Autodesk Fusion 360 part; units mm, degrees
(part 5 of 6)
  line L3180 (20.496389, 244.31625) -> (20.214167, 243.716528)
  line L3181 (20.214167, 243.716528) -> (20.0025, 243.116805)
  line L3182 (20.0025, 243.116805) -> (19.861389, 242.446528)
  line L3183 (19.861389, 242.446528) -> (19.790833, 241.811528)
  line L3184 (19.790833, 241.811528) -> (19.755556, 241.14125)
  line L3185 (19.755556, 241.14125) -> (19.790833, 240.50625)
  line L3186 (19.790833, 240.50625) -> (19.861389, 239.835972)
  line L3187 (19.861389, 239.835972) -> (20.0025, 239.200972)
  line L3188 (20.0025, 239.200972) -> (20.214167, 238.60125)
  line L3189 (20.214167, 238.60125) -> (20.496389, 237.96625)
  line L3190 (20.496389, 237.96625) -> (20.813889, 237.401805)
  line L3191 (20.813889, 237.401805) -> (21.166667, 236.872639)
  line L3192 (21.166667, 236.872639) -> (21.59, 236.37875)
  line L3193 (21.59, 236.37875) -> (22.048611, 235.884861)
  line L3194 (22.048611, 235.884861) -> (22.577778, 235.461528)
  line L3195 (22.577778, 235.461528) -> (23.106944, 235.10875)
  line L3196 (23.106944, 235.10875) -> (23.671389, 234.79125)
  line L3197 (23.671389, 234.79125) -> (24.271111, 234.509028)
  line L3198 (24.271111, 234.509028) -> (24.906111, 234.297361)
  line L3199 (24.906111, 234.297361) -> (25.541111, 234.15625)
  line L3200 (25.541111, 234.15625) -> (26.211389, 234.085694)
  line L3201 (26.211389, 234.085694) -> (26.846389, 234.050417)
  line L3202 (26.846389, 234.050417) -> (27.516667, 234.085694)
  line L3203 (27.516667, 234.085694) -> (28.151667, 234.15625)
  line L3204 (28.151667, 234.15625) -> (28.786667, 234.297361)
  line L3205 (28.786667, 234.297361) -> (29.421667, 234.509028)
  line L3206 (29.421667, 234.509028) -> (30.021389, 234.79125)
  line L3207 (30.021389, 234.79125) -> (30.585833, 235.10875)
  line L3208 (30.585833, 235.10875) -> (31.150278, 235.461528)
  line L3209 (31.150278, 235.461528) -> (31.644167, 235.884861)
  line L3210 (31.644167, 235.884861) -> (32.102778, 236.37875)
  line L3211 (32.102778, 236.37875) -> (32.526111, 236.872639)
  line L3212 (32.526111, 236.872639) -> (32.914167, 237.401805)
  line L3213 (32.914167, 237.401805) -> (33.231667, 237.96625)
  line L3214 (33.231667, 237.96625) -> (33.478611, 238.60125)
  line L3215 (33.478611, 238.60125) -> (33.690278, 239.200972)
  line L3216 (33.690278, 239.200972) -> (33.831389, 239.835972)
  line L3217 (33.831389, 239.835972) -> (33.937222, 240.50625)
  line L3218 (33.937222, 240.50625) -> (33.9725, 241.14125)
  line L3219 (28.116389, 289.577639) -> (28.116389, 289.471805)
  line L3220 (7.3025, 233.52125) -> (7.337778, 233.909305)
  line L3221 (31.326667, 225.760139) -> (29.845, 225.760139)
  line L3222 (9.419167, 223.467083) -> (9.454444, 223.220139)
  line L3223 (24.518056, 229.07625) -> (24.518056, 228.970417)
  line L3224 (24.518056, 228.970417) -> (24.482778, 228.899861)
  line L3225 (22.5425, 223.290694) -> (22.789444, 223.467083)
  line L3226 (39.722778, 242.72875) -> (39.863889, 242.446528)
  line L3227 (39.863889, 242.446528) -> (39.899167, 242.234861)
  line L3228 (39.511111, 242.834583) -> (39.616944, 242.799305)
  line L3229 (39.616944, 242.799305) -> (39.722778, 242.72875)
  line L3230 (24.765, 228.723472) -> (24.835556, 228.75875)
  line L3231 (24.835556, 228.75875) -> (24.870833, 228.794028)
  line L3232 (25.964444, 287.390417) -> (26.916944, 285.767639)
  line L3233 (22.789444, 223.467083) -> (22.965833, 223.643472)
  line L3234 (20.743333, 223.749305) -> (20.990278, 223.467083)
  line L3235 (23.318611, 230.593194) -> (23.565556, 230.487361)
  line L3236 (23.565556, 230.487361) -> (23.777222, 230.310972)
  line L3237 (23.777222, 230.310972) -> (23.918333, 229.993472)
  line L3238 (23.389167, 231.475139) -> (23.283333, 231.580972)
  line L3239 (23.283333, 231.580972) -> (23.106944, 231.61625)
  line L3240 (23.106944, 231.61625) -> (22.895278, 231.61625)
  line L3241 (40.005, 232.25125) -> (39.6875, 232.427639)
  line L3242 (16.721667, 291.024028) -> (16.474722, 291.094583)
  line L3243 (16.474722, 291.094583) -> (16.227778, 291.129861)
  line L3244 (38.205833, 233.168472) -> (38.205833, 236.343472)
  line L3245 (5.856111, 223.467083) -> (5.856111, 227.030139)
  line L3246 (5.856111, 227.030139) -> (5.856111, 227.17125)
  line L3247 (39.0525, 250.877917) -> (39.123056, 250.807361)
  line L3248 (39.123056, 250.807361) -> (39.158333, 250.772083)
  line L3249 (39.158333, 250.772083) -> (39.228889, 250.736805)
  line L3250 (39.228889, 250.736805) -> (39.299444, 250.736805)
  line L3251 (38.558611, 251.93625) -> (39.0525, 250.877917)
  line L3252 (39.440556, 265.306528) -> (39.37, 265.165417)
  line L3253 (38.205833, 236.343472) -> (38.205833, 236.449305)
  line L3254 (38.276389, 291.129861) -> (38.241111, 291.094583)
  line L3255 (40.005, 249.71375) -> (40.005, 251.93625)
  line L3256 (40.463611, 252.959305) -> (40.463611, 249.71375)
  line L3257 (30.938611, 291.059305) -> (30.903333, 291.129861)
  line L3258 (40.040278, 243.787083) -> (39.934444, 243.822361)
  line L3259 (39.828611, 241.917361) -> (39.899167, 242.234861)
  line L3260 (41.627778, 263.013472) -> (41.733611, 263.013472)
  line L3261 (41.380833, 263.295694) -> (41.416111, 263.119305)
  line L3262 (38.840833, 243.575417) -> (38.946667, 243.469583)
  line L3263 (27.340278, 291.129861) -> (27.305, 291.200417)
  line L3264 (17.250833, 222.549861) -> (22.154444, 222.549861)
  line L3265 (15.804444, 222.549861) -> (11.324167, 218.034306)
  line L3266 (40.287222, 262.378472) -> (40.181389, 262.801805)
  line L3267 (42.298056, 264.248194) -> (42.2275, 264.248194)
  line L3268 (37.994167, 291.588472) -> (38.064722, 291.553194)
  line L3269 (40.357778, 242.234861) -> (40.3225, 241.882083)
  line L3270 (20.778611, 225.548472) -> (20.743333, 225.26625)
  line L3271 (22.013333, 225.548472) -> (21.942778, 225.513194)
  line L3272 (22.754167, 225.548472) -> (22.154444, 225.548472)
  line L3273 (37.394444, 293.175972) -> (35.983333, 293.175972)
  line L3274 (24.835556, 285.59125) -> (24.906111, 285.626528)
  line L3275 (24.482778, 285.802917) -> (24.482778, 285.697083)
  line L3276 (35.983333, 293.175972) -> (35.983333, 291.588472)
  line L3277 (22.119167, 225.019305) -> (22.013333, 225.019305)
  line L3278 (39.193611, 276.736528) -> (39.264167, 276.665972)
  line L3279 (35.736389, 226.924305) -> (35.665833, 226.889028)
  line L3280 (39.698083, 284.522333) -> (36.935833, 281.745972)
  line L3281 (30.1625, 295.045694) -> (30.1625, 294.939861)
  line L3282 (38.205833, 242.164305) -> (38.241111, 242.340694)
  line L3283 (38.311667, 294.904583) -> (38.276389, 294.869305)
  line L3284 (37.711944, 223.220139) -> (37.676667, 223.290694)
  line L3285 (39.334722, 295.43375) -> (39.722778, 295.821805)
  line L3286 (26.881667, 252.077361) -> (26.387778, 252.077361)
  line L3287 (35.454167, 262.378472) -> (34.925, 264.212917)
  line L3288 (34.925, 264.212917) -> (34.360556, 262.378472)
  line L3289 (34.360556, 262.378472) -> (35.454167, 262.378472)
  line L3290 (32.102778, 227.347639) -> (32.138056, 227.277083)
  line L3291 (35.348333, 285.873472) -> (35.348333, 289.507083)
  line L3292 (15.663333, 286.86125) -> (16.051389, 286.825972)
  line L3293 (17.78, 290.283194) -> (17.603611, 290.459583)
  line L3294 (38.170556, 289.789305) -> (38.205833, 289.754028)
  line L3295 (21.096111, 289.789305) -> (20.955, 289.71875)
  line L3296 (20.955, 289.71875) -> (20.919722, 289.612917)
  line L3297 (20.073056, 290.283194) -> (25.611667, 295.821805)
  line L3298 (15.980833, 291.129861) -> (15.5575, 291.059305)
  line L3299 (16.227778, 291.129861) -> (15.980833, 291.129861)
  line L3300 (25.611667, 295.821805) -> (20.672778, 295.821805)
  line L3301 (17.603611, 290.459583) -> (17.391944, 290.635972)
  line L3302 (17.391944, 290.635972) -> (17.215556, 290.812361)
  line L3303 (29.068889, 231.722083) -> (28.998333, 231.651528)
  line L3304 (32.208611, 223.255417) -> (32.173333, 223.220139)
  line L3305 (37.641389, 293.669861) -> (37.711944, 293.599305)
  line L3306 (38.1, 252.924028) -> (38.135278, 253.100417)
  line L3307 (32.914167, 237.401805) -> (33.231667, 237.96625)
  line L3308 (33.231667, 237.96625) -> (33.478611, 238.60125)
  line L3309 (38.346944, 291.376805) -> (38.346944, 291.30625)
  line L3310 (31.891111, 227.382917) -> (32.102778, 227.347639)
  line L3311 (29.668611, 227.382917) -> (31.891111, 227.382917)
  line L3312 (32.208611, 227.100694) -> (32.173333, 226.994861)
  line L3313 (13.899444, 280.440694) -> (14.181667, 280.581805)
  line L3314 (31.538333, 280.440694) -> (31.785278, 280.264305)
  line L3315 (38.170556, 226.85375) -> (38.170556, 223.431805)
  line L3316 (38.205833, 233.027361) -> (38.205833, 233.168472)
  line L3317 (42.368611, 263.542639) -> (42.474444, 263.507361)
  line L3318 (19.861389, 239.835972) -> (20.0025, 239.200972)
  line L3319 (20.0025, 239.200972) -> (20.214167, 238.60125)
  line L3320 (32.208611, 223.467083) -> (32.243889, 223.396528)
  line L3321 (39.299444, 250.736805) -> (39.228889, 250.736805)
  line L3322 (20.955, 289.71875) -> (21.096111, 289.789305)
  line L3323 (21.096111, 289.789305) -> (21.2725, 289.824583)
  line L3324 (21.2725, 289.824583) -> (23.459722, 289.824583)
  line L3325 (22.471944, 229.71125) -> (22.436667, 229.817083)
  line L3326 (22.436667, 229.817083) -> (22.366111, 229.852361)
  line L3327 (38.629167, 243.116805) -> (38.488056, 243.257917)
  line L3328 (34.748611, 294.445972) -> (34.572222, 294.763472)
  line L3329 (19.05, 226.148194) -> (19.014722, 225.936528)
  line L3330 (22.013333, 225.548472) -> (22.154444, 225.548472)
  line L3331 (39.758056, 246.397639) -> (39.264167, 248.020417)
  line L3332 (39.264167, 248.020417) -> (38.770278, 246.397639)
  line L3333 (38.770278, 246.397639) -> (39.758056, 246.397639)
  line L3334 (23.847778, 246.750417) -> (24.412222, 247.032639)
  line L3335 (40.357778, 233.097917) -> (40.357778, 232.992083)
  line L3336 (27.410833, 291.094583) -> (27.340278, 291.129861)
  line L3337 (32.138056, 227.277083) -> (32.208611, 227.206528)
  line L3338 (40.463611, 253.100417) -> (40.463611, 252.959305)
  line L3339 (32.914167, 244.880694) -> (32.526111, 245.445139)
  line L3340 (32.526111, 245.445139) -> (32.102778, 245.939028)
  line L3341 (30.973889, 280.687639) -> (31.291389, 280.581805)
  line L3342 (39.123056, 265.694583) -> (39.228889, 265.694583)
  line L3343 (31.538333, 257.157361) -> (31.291389, 257.01625)
  line L3344 (32.138056, 226.924305) -> (32.102778, 226.889028)
  line L3345 (32.208611, 258.180417) -> (32.138056, 257.898194)
  line L3346 (14.181667, 257.01625) -> (13.899444, 257.157361)
  line L3347 (29.315833, 227.17125) -> (29.386389, 227.277083)
  line L3348 (31.291389, 225.26625) -> (29.845, 225.26625)
  line L3349 (39.017222, 237.33125) -> (39.017222, 237.190139)
  line L3350 (39.017222, 237.190139) -> (39.0525, 237.154861)
  line L3351 (33.901944, 286.261528) -> (34.043056, 286.402639)
  line L3352 (34.043056, 286.402639) -> (34.078333, 286.579028)
  line L3353 (20.990278, 238.707083) -> (21.2725, 238.177917)
  line L3354 (21.2725, 238.177917) -> (21.59, 237.613472)
  line L3355 (39.37, 244.457361) -> (39.123056, 244.457361)
  line L3356 (39.722778, 295.821805) -> (43.991389, 295.821805)
  line L3357 (29.950833, 253.488472) -> (29.280556, 252.112639)
  line L3358 (30.127222, 253.594305) -> (30.056667, 253.594305)
  line L3359 (28.398611, 233.450694) -> (29.104167, 233.591805)
  line L3360 (36.794722, 272.503194) -> (36.83, 272.57375)
  line L3361 (28.186944, 289.71875) -> (28.222222, 289.754028)
  line L3362 (35.806944, 289.507083) -> (35.806944, 288.166528)
  line L3363 (40.357778, 236.414028) -> (40.3225, 236.308194)
  line L3364 (36.83, 272.397361) -> (36.794722, 272.503194)
  line L3365 (13.6525, 257.369028) -> (13.476111, 257.615972)
  line L3366 (38.770278, 241.77625) -> (38.911389, 241.635139)
  line L3367 (35.736389, 289.754028) -> (35.806944, 289.648194)
  line L3368 (40.393056, 253.170972) -> (40.463611, 253.100417)
  line L3369 (29.280556, 252.112639) -> (29.950833, 253.488472)
  line L3370 (38.276389, 232.921528) -> (38.382222, 232.88625)
  line L3371 (38.382222, 232.88625) -> (38.488056, 232.88625)
  line L3372 (38.205833, 236.343472) -> (38.205833, 233.168472)
  line L3373 (38.523333, 236.660972) -> (38.382222, 236.625694)
  line L3374 (38.382222, 236.625694) -> (38.241111, 236.555139)
  line L3375 (29.986111, 230.381528) -> (29.986111, 229.111528)
  line L3376 (20.496389, 241.14125) -> (20.531667, 240.541528)
  line L3377 (20.531667, 240.541528) -> (20.6375, 239.906528)
  line L3378 (37.958889, 289.789305) -> (38.064722, 289.824583)
  line L3379 (30.832778, 294.975139) -> (30.832778, 291.341528)
  line L3380 (31.538333, 225.724861) -> (31.608889, 225.689583)
  line L3381 (14.499167, 280.687639) -> (14.781389, 280.722917)
  line L3382 (1.446389, 284.709305) -> (1.446389, 284.391805)
  line L3383 (5.150556, 292.999583) -> (1.446389, 284.709305)
  line L3384 (21.942778, 245.198194) -> (22.366111, 245.656805)
  line L3385 (40.3225, 228.970417) -> (40.3225, 228.899861)
  line L3386 (40.3225, 228.899861) -> (40.251944, 228.829305)
  line L3387 (40.251944, 228.829305) -> (40.181389, 228.75875)
  line L3388 (40.181389, 228.75875) -> (40.075556, 228.75875)
  line L3389 (40.075556, 228.75875) -> (39.969722, 228.75875)
  line L3390 (39.969722, 228.75875) -> (39.934444, 228.794028)
  line L3391 (39.934444, 228.794028) -> (39.899167, 228.864583)
  line L3392 (39.899167, 228.864583) -> (39.0525, 230.310972)
  line L3393 (39.0525, 230.310972) -> (38.735, 230.310972)
  line L3394 (38.735, 230.310972) -> (38.735, 229.040972)
  line L3395 (38.735, 229.040972) -> (38.735, 228.935139)
  line L3396 (38.735, 228.935139) -> (38.699722, 228.829305)
  line L3397 (38.699722, 228.829305) -> (38.664444, 228.75875)
  line L3398 (38.664444, 228.75875) -> (38.593889, 228.75875)
  line L3399 (38.593889, 228.75875) -> (38.488056, 228.723472)
  line L3400 (38.488056, 228.723472) -> (38.4175, 228.75875)
  line L3401 (38.4175, 228.75875) -> (38.311667, 228.794028)
  line L3402 (38.311667, 228.794028) -> (38.276389, 228.864583)
  line L3403 (38.276389, 228.864583) -> (38.276389, 228.899861)
  line L3404 (38.276389, 228.899861) -> (38.276389, 229.040972)
  line L3405 (38.276389, 229.040972) -> (38.276389, 232.180694)
  line L3406 (38.276389, 232.180694) -> (38.276389, 232.286528)
  line L3407 (38.276389, 232.286528) -> (38.311667, 232.392361)
  line L3408 (38.311667, 232.392361) -> (38.452778, 232.498194)
  line L3409 (38.452778, 232.498194) -> (38.593889, 232.498194)
  line L3410 (38.593889, 232.498194) -> (39.334722, 232.498194)
  line L3411 (39.334722, 232.498194) -> (39.6875, 232.427639)
  line L3412 (39.6875, 232.427639) -> (40.005, 232.25125)
  line L3413 (40.005, 232.25125) -> (40.216667, 231.863194)
  line L3414 (40.216667, 231.863194) -> (40.3225, 231.404583)
  line L3415 (40.3225, 231.404583) -> (40.287222, 231.122361)
  line L3416 (40.287222, 231.122361) -> (40.181389, 230.840139)
  line L3417 (40.181389, 230.840139) -> (39.934444, 230.522639)
  line L3418 (39.934444, 230.522639) -> (39.616944, 230.34625)
  line L3419 (39.616944, 230.34625) -> (39.581667, 230.310972)
  line L3420 (39.581667, 230.310972) -> (40.216667, 229.182083)
  line L3421 (40.216667, 229.182083) -> (40.251944, 229.146805)
  line L3422 (40.251944, 229.146805) -> (40.287222, 229.07625)
  line L3423 (40.287222, 229.07625) -> (40.3225, 229.040972)
  line L3424 (40.3225, 229.040972) -> (40.3225, 228.970417)
  line L3425 (38.488056, 232.88625) -> (38.382222, 232.88625)
  line L3426 (38.382222, 232.88625) -> (38.276389, 232.921528)
  line L3427 (13.229167, 279.452917) -> (13.335, 279.735139)
  line L3428 (15.24, 225.760139) -> (15.451667, 225.724861)
  line L3429 (40.040278, 232.88625) -> (38.488056, 232.88625)
  line L3430 (42.403889, 264.283472) -> (42.298056, 264.248194)
  line L3431 (14.181667, 280.581805) -> (14.499167, 280.687639)
  line L3432 (15.522222, 225.689583) -> (15.5575, 225.58375)
  line L3433 (31.150278, 235.461528) -> (31.644167, 235.884861)
  line L3434 (31.644167, 235.884861) -> (32.102778, 236.37875)
  line L3435 (27.410833, 285.661805) -> (27.305, 285.59125)
  line L3436 (21.872222, 225.054583) -> (21.801667, 225.125139)
  line L3437 (32.949444, 243.010972) -> (33.090556, 242.375972)
  line L3438 (13.6525, 280.264305) -> (13.899444, 280.440694)
  line L3439 (32.0675, 223.643472) -> (32.173333, 223.537639)
  line L3440 (35.418889, 285.626528) -> (35.348333, 285.732361)
  line L3441 (35.806944, 287.707917) -> (35.806944, 285.873472)
  line L3442 (41.169167, 261.814028) -> (41.310278, 261.708194)
  line L3443 (39.264167, 248.020417) -> (39.758056, 246.397639)
  line L3444 (39.405278, 244.95125) -> (39.440556, 244.95125)
  line L3445 (22.789444, 226.254028) -> (22.718889, 226.289305)
  line L3446 (20.849167, 225.830694) -> (21.060833, 226.254028)
  line L3447 (21.201944, 223.99625) -> (20.990278, 224.31375)
  line L3448 (20.990278, 224.31375) -> (20.849167, 224.666528)
  line L3449 (28.786667, 247.985139) -> (28.151667, 248.161528)
  line L3450 (28.151667, 248.161528) -> (27.516667, 248.232083)
  line L3451 (39.264167, 276.524861) -> (39.228889, 276.419028)
  line L3452 (39.228889, 250.736805) -> (39.158333, 250.772083)
  line L3453 (33.725556, 284.885694) -> (30.585833, 281.745972)
  line L3454 (38.311667, 232.392361) -> (38.276389, 232.286528)
  line L3455 (37.641389, 293.669861) -> (37.429722, 293.705139)
  line L3456 (37.394444, 293.175972) -> (37.641389, 293.21125)
  line L3457 (37.641389, 293.21125) -> (37.711944, 293.246528)
  line L3458 (31.467778, 228.829305) -> (31.4325, 228.75875)
  line L3459 (13.899444, 289.048472) -> (13.934722, 288.695694)
  line L3460 (13.934722, 288.695694) -> (14.005278, 288.307639)
  line L3461 (30.021389, 247.526528) -> (29.421667, 247.773472)
  line L3462 (29.421667, 247.773472) -> (28.786667, 247.985139)
  line L3463 (19.332222, 226.85375) -> (19.085278, 227.135972)
  line L3464 (19.085278, 227.135972) -> (18.697222, 227.312361)
  line L3465 (39.6875, 241.211805) -> (39.969722, 241.352917)
  line L3466 (39.969722, 241.352917) -> (40.181389, 241.564583)
  line L3467 (40.181389, 241.564583) -> (40.3225, 241.882083)
  line L3468 (40.3225, 241.882083) -> (40.357778, 242.234861)
  line L3469 (8.713611, 223.220139) -> (8.748889, 223.255417)
  line L3470 (8.748889, 223.255417) -> (8.748889, 223.396528)
  line L3471 (17.250833, 222.549861) -> (22.154444, 222.549861)
  line L3472 (23.600833, 222.549861) -> (28.504444, 222.549861)
  line L3473 (29.950833, 222.549861) -> (31.855833, 222.549861)
  line L3474 (38.135278, 249.537361) -> (38.1, 249.749028)
  line L3475 (8.396111, 223.114305) -> (8.643056, 223.149583)
  line L3476 (8.643056, 223.149583) -> (8.713611, 223.220139)
  line L3477 (30.903333, 291.129861) -> (30.832778, 291.165139)
  line L3478 (24.906111, 247.985139) -> (24.271111, 247.773472)
  line L3479 (24.271111, 247.773472) -> (23.671389, 247.526528)
  line L3480 (40.3225, 241.882083) -> (40.181389, 241.564583)
  line L3481 (29.315833, 223.467083) -> (29.315833, 227.030139)
  line L3482 (40.357778, 233.168472) -> (40.357778, 233.097917)
  line L3483 (17.321389, 226.85375) -> (18.273889, 226.85375)
  line L3484 (17.321389, 225.407361) -> (17.321389, 226.85375)
  line L3485 (11.43, 232.639305) -> (11.535833, 232.992083)
  line L3486 (11.535833, 232.992083) -> (11.606389, 233.344861)
  line L3487 (23.988889, 229.640694) -> (23.918333, 229.993472)
  line L3488 (28.716111, 230.628472) -> (28.680833, 230.699028)
  line L3489 (28.680833, 230.699028) -> (28.645556, 230.734305)
  line L3490 (28.645556, 230.734305) -> (28.469167, 230.769583)
  line L3491 (27.093333, 251.689305) -> (27.128611, 251.724583)
  line L3492 (27.693056, 250.701528) -> (27.093333, 251.689305)
  line L3493 (27.375556, 284.885694) -> (27.199167, 284.885694)
  line L3494 (38.170556, 289.789305) -> (38.064722, 289.824583)
  line L3495 (38.276389, 285.873472) -> (38.276389, 289.507083)
  line L3496 (38.064722, 285.555972) -> (38.170556, 285.59125)
  line L3497 (31.573611, 247.455972) -> (31.009167, 247.844028)
  line L3498 (31.009167, 247.844028) -> (30.374167, 248.196805)
  line L3499 (8.713611, 223.537639) -> (8.5725, 223.643472)
  line L3500 (33.090556, 242.375972) -> (33.161111, 241.77625)
  line L3501 (32.173333, 226.994861) -> (32.138056, 226.924305)
  line L3502 (25.611667, 247.385417) -> (26.246667, 247.455972)
  line L3503 (19.508611, 225.760139) -> (19.579167, 226.148194)
  line L3504 (19.473333, 223.608194) -> (18.520833, 224.913472)
  line L3505 (11.606389, 233.344861) -> (11.535833, 232.992083)
  line L3506 (32.243889, 223.396528) -> (32.208611, 223.255417)
  line L3507 (38.064722, 223.149583) -> (37.923611, 223.114305)
  line L3508 (26.281944, 287.884305) -> (27.093333, 289.365972)
  line L3509 (29.5275, 227.347639) -> (29.668611, 227.382917)
  line L3510 (28.645556, 230.381528) -> (28.433889, 230.381528)
  line L3511 (34.219444, 288.730972) -> (34.29, 288.695694)
  line L3512 (34.29, 288.695694) -> (34.360556, 288.695694)
  line L3513 (27.340278, 228.723472) -> (27.410833, 228.723472)
  line L3514 (29.068889, 231.792639) -> (29.033611, 231.898472)
  line L3515 (29.033611, 231.898472) -> (28.963056, 231.969028)
  line L3516 (28.963056, 231.969028) -> (28.821944, 232.004305)
  line L3517 (28.292778, 253.488472) -> (28.328056, 253.559028)
  line L3518 (22.401389, 223.819861) -> (22.507222, 223.960972)
  line L3519 (31.361944, 236.660972) -> (30.868056, 236.237639)
  line L3520 (27.234444, 231.93375) -> (27.199167, 231.827917)
  line L3521 (27.199167, 231.827917) -> (27.199167, 231.722083)
  line L3522 (28.821944, 232.004305) -> (27.481389, 232.004305)
  line L3523 (13.193889, 279.135417) -> (13.229167, 279.452917)
  line L3524 (18.803056, 226.677361) -> (18.944167, 226.500972)
  line L3525 (18.944167, 226.500972) -> (19.014722, 226.324583)
  line L3526 (32.737778, 243.575417) -> (32.455556, 244.139861)
  line L3527 (32.455556, 244.139861) -> (32.138056, 244.669028)
  line L3528 (13.476111, 280.017361) -> (13.6525, 280.264305)
  line L3529 (32.984722, 227.312361) -> (33.231667, 227.382917)
  line L3530 (35.771667, 227.100694) -> (35.771667, 227.030139)
  line L3531 (39.37, 265.165417) -> (37.500278, 261.284861)
  line L3532 (29.598056, 228.970417) -> (29.598056, 231.757361)
  line L3533 (28.222222, 227.312361) -> (28.292778, 227.347639)
  line L3534 (16.051389, 226.924305) -> (16.016111, 226.889028)
  line L3535 (32.138056, 279.735139) -> (32.208611, 279.452917)
  line L3536 (8.607778, 227.347639) -> (8.396111, 227.382917)
  line L3537 (23.777222, 285.626528) -> (23.8125, 285.697083)
  line L3538 (21.237222, 285.555972) -> (23.459722, 285.555972)
  line L3539 (29.386389, 227.277083) -> (29.5275, 227.347639)
  line L3540 (38.770278, 244.210417) -> (38.911389, 244.386805)
  line L3541 (30.973889, 256.945694) -> (30.656389, 256.910417)
  line L3542 (41.768889, 261.708194) -> (41.557222, 261.672917)
  line L3543 (28.081111, 234.932361) -> (28.716111, 235.073472)
  line L3544 (28.716111, 235.073472) -> (29.280556, 235.285139)
  line L3545 (38.593889, 242.41125) -> (38.664444, 242.305417)
  line L3546 (25.294167, 289.612917) -> (25.964444, 288.44875)
  line L3547 (32.208611, 279.452917) -> (32.243889, 279.135417)
  line L3548 (31.538333, 225.301528) -> (31.291389, 225.26625)
  line L3549 (27.798889, 294.763472) -> (27.798889, 293.705139)
  line L3550 (37.676667, 226.85375) -> (36.794722, 226.85375)
  line L3551 (40.3225, 232.956805) -> (40.287222, 232.921528)
  line L3552 (32.102778, 223.149583) -> (31.855833, 223.114305)
  line L3553 (39.793333, 244.845417) -> (39.616944, 244.915972)
  line L3554 (28.680833, 227.135972) -> (28.680833, 227.030139)
  line L3555 (1.446389, 284.391805) -> (1.446389, 284.709305)
  line L3556 (21.2725, 238.177917) -> (20.990278, 238.707083)
  line L3557 (42.545, 263.189861) -> (42.545, 262.202083)
  line L3558 (21.942778, 237.119583) -> (21.59, 237.613472)
  line L3559 (32.455556, 244.139861) -> (32.737778, 243.575417)
  line L3560 (36.794722, 226.85375) -> (36.583056, 226.889028)
  line L3561 (13.758333, 226.85375) -> (13.758333, 225.760139)
  line L3562 (28.010556, 224.137361) -> (28.116389, 224.419583)
  line L3563 (36.300833, 222.549861) -> (37.923611, 222.549861)
  line L3564 (37.923611, 222.549861) -> (41.204444, 222.549861)
  line L3565 (27.6225, 230.381528) -> (27.6225, 228.970417)
  line L3566 (28.610278, 227.312361) -> (28.645556, 227.206528)
  line L3567 (22.577778, 225.019305) -> (22.119167, 225.019305)
  line L3568 (13.758333, 225.760139) -> (15.24, 225.760139)
  line L3569 (38.382222, 243.434305) -> (38.488056, 243.257917)
  line L3570 (39.405278, 241.14125) -> (39.123056, 241.14125)
  line L3571 (34.466389, 289.330694) -> (34.219444, 289.542361)
  line L3572 (34.219444, 289.542361) -> (33.901944, 289.71875)
  line L3573 (22.824722, 246.080139) -> (23.318611, 246.432917)
  line L3574 (28.292778, 250.384028) -> (28.2575, 250.560417)
  line L3575 (22.154444, 231.157639) -> (22.189722, 230.910694)
  line L3576 (22.189722, 230.910694) -> (22.260278, 230.699028)
  line L3577 (32.208611, 289.119028) -> (32.596667, 289.542361)
  line L3578 (32.596667, 289.542361) -> (32.949444, 289.71875)
  line L3579 (32.737778, 243.575417) -> (32.949444, 243.010972)
  line L3580 (29.5275, 223.114305) -> (29.421667, 223.184861)
  line L3581 (20.6375, 239.906528) -> (20.531667, 240.541528)
  line L3582 (31.996944, 280.017361) -> (32.138056, 279.735139)
  line L3583 (31.785278, 280.264305) -> (31.996944, 280.017361)
  line L3584 (29.315833, 227.030139) -> (29.315833, 227.17125)
  line L3585 (13.476111, 280.017361) -> (13.335, 279.735139)
  line L3586 (13.335, 279.735139) -> (13.229167, 279.452917)
  line L3587 (13.229167, 279.452917) -> (13.193889, 279.135417)
  line L3588 (30.656389, 280.722917) -> (14.781389, 280.722917)
  line L3589 (39.722778, 242.72875) -> (39.616944, 242.799305)
  line L3590 (35.806944, 288.166528) -> (37.817778, 288.166528)
  line L3591 (16.086667, 227.277083) -> (16.121944, 227.206528)
  line L3592 (32.173333, 223.220139) -> (32.102778, 223.149583)
  line L3593 (29.668611, 223.114305) -> (29.5275, 223.114305)
  line L3594 (32.208611, 227.135972) -> (32.208611, 227.100694)
  line L3595 (31.855833, 223.114305) -> (29.668611, 223.114305)
  line L3596 (41.521944, 263.507361) -> (41.627778, 263.542639)
  line L3597 (41.416111, 263.119305) -> (41.380833, 263.295694)
  line L3598 (39.37, 226.994861) -> (39.334722, 226.924305)
  line L3599 (35.489444, 289.789305) -> (35.56, 289.824583)
  line L3600 (29.245278, 293.705139) -> (29.386389, 293.705139)
  line L3601 (31.785278, 287.249305) -> (31.75, 287.672639)
  line L3602 (31.75, 287.672639) -> (31.785278, 288.13125)
  line L3603 (35.665833, 285.555972) -> (35.595278, 285.555972)
  line L3604 (38.170556, 223.255417) -> (38.064722, 223.149583)
  line L3605 (29.492222, 293.634583) -> (29.5275, 293.599305)
  line L3606 (40.287222, 240.400417) -> (40.181389, 240.329861)
  line L3607 (26.140833, 224.878194) -> (26.176111, 224.772361)
  line L3608 (27.551944, 228.75875) -> (27.516667, 228.723472)
  line L3609 (29.739167, 232.004305) -> (29.845, 232.004305)
  line L3610 (6.0325, 227.347639) -> (6.208889, 227.382917)
  line L3611 (6.208889, 227.382917) -> (8.396111, 227.382917)
  line L3612 (40.3225, 232.956805) -> (40.357778, 232.992083)
  line L3613 (40.357778, 232.992083) -> (40.357778, 233.097917)
  line L3614 (38.488056, 232.88625) -> (40.040278, 232.88625)
  line L3615 (24.553333, 285.626528) -> (24.482778, 285.697083)
  line L3616 (29.068889, 231.792639) -> (29.068889, 231.722083)
  line L3617 (34.748611, 291.482639) -> (34.713333, 291.517917)
  line L3618 (34.819167, 291.30625) -> (34.783889, 291.412083)
  line L3619 (34.783889, 291.412083) -> (34.748611, 291.482639)
  line L3620 (38.735, 230.310972) -> (39.0525, 230.310972)
  line L3621 (38.735, 229.040972) -> (38.735, 230.310972)
  line L3622 (39.158333, 237.01375) -> (39.087778, 237.084305)
  line L3623 (38.770278, 241.211805) -> (38.488056, 241.388194)
  line L3624 (15.204722, 225.26625) -> (13.758333, 225.26625)
  line L3625 (25.999722, 229.675972) -> (25.576389, 231.087083)
  line L3626 (25.576389, 231.087083) -> (25.153056, 229.675972)
  line L3627 (25.153056, 229.675972) -> (25.999722, 229.675972)
  line L3628 (14.640278, 287.355139) -> (14.957778, 287.108194)
  line L3629 (32.385, 291.059305) -> (32.455556, 291.094583)
  line L3630 (32.455556, 291.094583) -> (32.490833, 291.165139)
  line L3631 (21.343056, 246.785694) -> (20.884444, 246.291805)
  line L3632 (20.884444, 246.291805) -> (20.461111, 245.727361)
  line L3633 (20.461111, 245.727361) -> (20.073056, 245.127639)
  line L3634 (35.806944, 288.166528) -> (35.806944, 289.507083)
  line L3635 (37.817778, 288.166528) -> (35.806944, 288.166528)
  line L3636 (25.505833, 232.004305) -> (25.435278, 231.969028)
  line L3637 (25.435278, 231.969028) -> (25.4, 231.93375)
  line L3638 (28.927778, 231.61625) -> (28.821944, 231.61625)
  line L3639 (34.536944, 287.919583) -> (34.6075, 287.778472)
  line L3640 (39.334722, 289.08375) -> (39.334722, 284.885694)
  line L3641 (27.093333, 289.365972) -> (26.281944, 287.884305)
  line L3642 (27.693056, 253.029861) -> (27.481389, 253.382639)
  line L3643 (27.481389, 253.382639) -> (27.199167, 253.559028)
  line L3644 (40.216667, 243.892917) -> (40.251944, 243.963472)
  line L3645 (40.251944, 243.963472) -> (40.287222, 244.034028)
  line L3646 (39.828611, 243.892917) -> (39.899167, 243.857639)
  line L3647 (39.899167, 243.857639) -> (39.934444, 243.822361)
  line L3648 (33.655, 287.460972) -> (34.113611, 287.460972)
  line L3649 (33.408056, 287.49625) -> (33.478611, 287.460972)
  line L3650 (31.926389, 288.589861) -> (31.785278, 288.13125)
  line L3651 (31.785278, 288.13125) -> (31.75, 287.672639)
  line L3652 (41.733611, 263.013472) -> (41.627778, 263.013472)
  line L3653 (15.663333, 286.86125) -> (16.051389, 286.825972)
  line L3654 (26.035, 224.984028) -> (26.105556, 224.94875)
  line L3655 (13.758333, 226.85375) -> (15.769167, 226.85375)
  line L3656 (13.758333, 225.760139) -> (13.758333, 226.85375)
  line L3657 (15.24, 225.760139) -> (13.758333, 225.760139)
  line L3658 (13.193889, 279.135417) -> (13.193889, 258.497917)
  line L3659 (17.674167, 218.034306) -> (12.735278, 218.034306)
  line L3660 (12.735278, 218.034306) -> (17.250833, 222.549861)
  line L3661 (21.448889, 286.085139) -> (21.448889, 287.707917)
  line L3662 (27.551944, 250.313472) -> (27.6225, 250.34875)
  line L3663 (27.6225, 250.34875) -> (27.728333, 250.384028)
  line L3664 (36.477222, 227.135972) -> (36.477222, 227.241805)
  line L3665 (20.214167, 238.60125) -> (20.496389, 237.96625)
  line L3666 (20.496389, 237.96625) -> (20.813889, 237.401805)
  line L3667 (28.292778, 250.384028) -> (28.328056, 250.34875)
  line L3668 (28.328056, 250.34875) -> (28.363333, 250.313472)
  line L3669 (38.205833, 295.257361) -> (37.994167, 295.292639)
  line L3670 (34.783889, 294.057917) -> (34.748611, 294.445972)
  line L3671 (38.523333, 253.065139) -> (38.523333, 253.135694)
  line L3672 (23.636111, 233.979861) -> (24.306389, 233.697639)
  line L3673 (24.306389, 233.697639) -> (24.976667, 233.52125)
  line L3674 (24.976667, 233.52125) -> (25.646944, 233.380139)
  line L3675 (33.443333, 289.295417) -> (33.655, 289.260139)
  line L3676 (33.655, 289.260139) -> (33.866667, 289.154305)
  line L3677 (10.900833, 222.549861) -> (6.385278, 218.034306)
  line L3678 (4.974167, 218.034306) -> (6.385278, 218.034306)
  line L3679 (27.657778, 295.292639) -> (29.809722, 295.292639)
  line L3680 (40.463611, 245.374583) -> (40.498889, 245.445139)
  line L3681 (40.498889, 245.445139) -> (40.534167, 245.515694)
  line L3682 (38.276389, 243.928194) -> (38.311667, 243.68125)
  line L3683 (38.311667, 243.68125) -> (38.382222, 243.434305)
  line L3684 (38.488056, 228.723472) -> (38.593889, 228.75875)
  line L3685 (38.593889, 228.75875) -> (38.664444, 228.75875)
  line L3686 (38.664444, 228.75875) -> (38.699722, 228.829305)
  line L3687 (38.699722, 228.829305) -> (38.735, 228.935139)
  line L3688 (38.735, 228.935139) -> (38.735, 229.040972)
  line L3689 (15.875, 223.643472) -> (15.980833, 223.643472)
  line L3690 (5.185833, 281.745972) -> (1.446389, 281.745972)
  line L3691 (23.142222, 229.111528) -> (22.895278, 229.111528)
  line L3692 (23.389167, 229.182083) -> (23.248056, 229.111528)
  line L3693 (23.318611, 235.884861) -> (23.847778, 235.567361)
  line L3694 (23.847778, 235.567361) -> (24.412222, 235.285139)
  line L3695 (22.824722, 231.580972) -> (22.895278, 231.61625)
  line L3696 (22.5425, 231.157639) -> (22.613056, 231.369305)
  line L3697 (40.110833, 242.975694) -> (40.287222, 242.622917)
  line L3698 (11.006667, 232.039583) -> (11.253611, 232.321805)
  line L3699 (11.253611, 232.321805) -> (11.43, 232.639305)
  line L3700 (27.446111, 250.34875) -> (27.551944, 250.313472)
  line L3701 (26.634722, 251.689305) -> (27.375556, 250.419305)
  line L3702 (26.3525, 295.151528) -> (21.484167, 290.283194)
  line L3703 (43.991389, 293.740417) -> (43.991389, 295.186805)
  line L3704 (39.934444, 235.073472) -> (39.934444, 235.002917)
  line L3705 (37.7825, 223.149583) -> (37.711944, 223.220139)
  line L3706 (23.1775, 288.13125) -> (23.106944, 288.166528)
  line L3707 (23.106944, 288.166528) -> (22.895278, 288.201805)
  line L3708 (5.150556, 292.999583) -> (7.972778, 295.821805)
  line L3709 (12.594167, 227.100694) -> (12.594167, 223.431805)
  line L3710 (37.041667, 261.284861) -> (37.112222, 261.179028)
  line L3711 (37.112222, 261.179028) -> (37.182778, 261.14375)
  line L3712 (11.1125, 224.595972) -> (10.971389, 224.595972)
  line L3713 (26.105556, 224.94875) -> (26.035, 224.984028)
  line L3714 (26.035, 224.984028) -> (25.893889, 225.019305)
  line L3715 (26.176111, 224.63125) -> (26.176111, 224.772361)
  line L3716 (27.410833, 291.094583) -> (27.551944, 291.059305)
  line L3717 (27.269722, 291.376805) -> (27.269722, 291.270972)
  line L3718 (27.269722, 291.270972) -> (27.305, 291.200417)
  line L3719 (27.269722, 294.939861) -> (27.269722, 291.376805)
  line L3720 (36.477222, 227.030139) -> (36.5125, 226.959583)
  line L3721 (36.5125, 226.959583) -> (36.583056, 226.889028)
  line L3722 (36.583056, 226.889028) -> (36.794722, 226.85375)
  line L3723 (32.138056, 244.669028) -> (32.455556, 244.139861)
  line L3724 (39.0525, 248.972917) -> (39.0525, 248.902361)
  line L3725 (39.511111, 248.867083) -> (39.475833, 248.972917)
  line L3726 (39.475833, 248.972917) -> (39.405278, 249.043472)
  line L3727 (39.405278, 249.043472) -> (39.334722, 249.07875)
  line L3728 (27.340278, 252.641805) -> (27.305, 252.359583)
  line L3729 (29.809722, 295.292639) -> (30.021389, 295.257361)
  line L3730 (34.29, 285.90875) -> (34.078333, 285.732361)
  line L3731 (34.078333, 285.732361) -> (33.760833, 285.626528)
  line L3732 (1.446389, 220.891806) -> (1.446389, 219.445417)
  line L3733 (1.446389, 220.891806) -> (3.104444, 222.549861)
  line L3734 (9.525, 223.149583) -> (9.666111, 223.114305)
  line L3735 (9.419167, 227.030139) -> (9.419167, 223.467083)
  line L3736 (9.666111, 227.347639) -> (9.595556, 227.347639)
  line L3737 (10.724444, 224.772361) -> (9.913056, 226.112917)
  line L3738 (32.949444, 289.71875) -> (33.408056, 289.824583)
  line L3739 (33.408056, 289.824583) -> (33.690278, 289.789305)
  line L3740 (38.276389, 232.286528) -> (38.276389, 232.180694)
  line L3741 (39.334722, 232.498194) -> (38.593889, 232.498194)
  line L3742 (31.785278, 218.034306) -> (36.300833, 222.549861)
  line L3743 (1.446389, 222.549861) -> (1.446389, 220.891806)
  line L3744 (35.701111, 272.291528) -> (35.771667, 272.25625)
  line L3745 (35.771667, 272.25625) -> (35.842222, 272.25625)
  line L3746 (35.418889, 272.961805) -> (35.595278, 272.432639)
  line L3747 (33.549167, 261.249583) -> (33.619722, 261.179028)
  line L3748 (26.246667, 228.864583) -> (26.281944, 228.794028)
  line L3749 (26.281944, 228.794028) -> (26.3525, 228.723472)
  line L3750 (38.276389, 253.20625) -> (38.346944, 253.20625)
  line L3751 (26.387778, 253.20625) -> (26.916944, 253.20625)
  line L3752 (27.340278, 252.641805) -> (27.305, 252.359583)
  line L3753 (27.305, 252.359583) -> (27.199167, 252.183194)
  line L3754 (27.128611, 253.135694) -> (27.234444, 253.029861)
  line L3755 (13.299722, 227.277083) -> (13.264444, 227.17125)
  line L3756 (13.264444, 227.17125) -> (13.229167, 227.030139)
  line L3757 (27.410833, 228.723472) -> (27.516667, 228.723472)
  line L3758 (11.535833, 281.745972) -> (6.596944, 281.745972)
  line L3759 (36.265556, 261.214305) -> (36.300833, 261.284861)
  line L3760 (12.523611, 223.220139) -> (12.453056, 223.149583)
  line L3761 (37.676667, 223.467083) -> (37.676667, 226.85375)
  line L3762 (31.467778, 231.827917) -> (31.467778, 231.722083)
  line L3763 (39.405278, 227.100694) -> (39.37, 227.241805)
  line L3764 (39.37, 227.241805) -> (39.264167, 227.312361)
  line L3765 (39.264167, 227.312361) -> (39.0525, 227.382917)
  line L3766 (26.140833, 229.252639) -> (26.246667, 228.864583)
  line L3767 (25.011944, 229.252639) -> (26.140833, 229.252639)
  line L3768 (30.938611, 289.754028) -> (31.009167, 289.683472)
  line L3769 (22.789444, 229.111528) -> (22.895278, 229.111528)
  line L3770 (22.895278, 229.111528) -> (23.142222, 229.111528)
  line L3771 (23.142222, 229.111528) -> (23.248056, 229.111528)
  line L3772 (23.248056, 229.111528) -> (23.142222, 229.111528)
  line L3773 (23.565556, 229.640694) -> (23.530278, 229.358472)
  line L3774 (40.005, 244.669028) -> (40.146111, 244.457361)
  line L3775 (22.401389, 223.819861) -> (22.225, 223.714028)
  line L3776 (22.225, 223.714028) -> (21.942778, 223.643472)
  line L3777 (26.740556, 223.749305) -> (27.163889, 223.643472)
  line L3778 (34.572222, 294.763472) -> (34.325278, 295.045694)
  line L3779 (34.325278, 295.045694) -> (33.901944, 295.222083)
  line L3780 (33.901944, 295.222083) -> (33.478611, 295.292639)
  line L3781 (22.366111, 229.852361) -> (22.295556, 229.852361)
  line L3782 (22.895278, 229.111528) -> (22.789444, 229.111528)
  line L3783 (40.781111, 273.490972) -> (41.345556, 275.325417)
  line L3784 (40.675278, 263.260417) -> (40.710556, 263.754305)
  line L3785 (40.710556, 263.754305) -> (40.851667, 264.212917)
  line L3786 (40.851667, 264.212917) -> (40.992778, 264.424583)
  line L3787 (38.452778, 242.481805) -> (38.523333, 242.481805)
  line L3788 (16.721667, 291.024028) -> (16.474722, 291.094583)
  line L3789 (16.474722, 291.094583) -> (16.227778, 291.129861)
  line L3790 (41.874722, 264.671528) -> (42.051111, 264.424583)
  line L3791 (41.733611, 264.812639) -> (41.874722, 264.671528)
  line L3792 (22.401389, 227.277083) -> (22.154444, 227.347639)
  line L3793 (22.154444, 227.347639) -> (21.9075, 227.382917)
  line L3794 (11.183056, 224.666528) -> (11.1125, 224.595972)
  line L3795 (40.287222, 232.921528) -> (40.040278, 232.88625)
  line L3796 (32.596667, 288.695694) -> (32.773056, 288.942639)
  line L3797 (32.773056, 288.942639) -> (32.984722, 289.154305)
  line L3798 (40.251944, 240.753194) -> (40.075556, 240.788472)
  line L3799 (40.040278, 236.167083) -> (40.181389, 236.202361)
  line L3800 (40.181389, 236.202361) -> (40.287222, 236.237639)
  line L3801 (23.353889, 230.134583) -> (23.424444, 230.064028)
  line L3802 (22.789444, 230.275694) -> (23.212778, 230.169861)
  line L3803 (15.310556, 286.967083) -> (15.663333, 286.86125)
  line L3804 (38.276389, 232.921528) -> (38.205833, 233.027361)
  line L3805 (28.539722, 250.313472) -> (28.610278, 250.34875)
  line L3806 (28.610278, 250.34875) -> (28.645556, 250.384028)
  line L3807 (31.644167, 225.58375) -> (31.644167, 225.513194)
  line L3808 (42.051111, 263.013472) -> (42.051111, 262.343194)
  line L3809 (41.733611, 263.013472) -> (42.051111, 263.013472)
  line L3810 (28.716111, 230.452083) -> (28.680833, 230.416805)
  line L3811 (40.075556, 236.660972) -> (40.251944, 236.625694)
  line L3812 (38.1, 294.763472) -> (37.958889, 294.763472)
  line L3813 (40.216667, 244.280972) -> (40.287222, 244.034028)
  line L3814 (38.876111, 276.736528) -> (38.946667, 276.807083)
  line L3815 (26.811111, 289.789305) -> (26.740556, 289.754028)
  line L3816 (27.199167, 289.577639) -> (27.163889, 289.683472)
  line L3817 (28.680833, 230.416805) -> (28.645556, 230.381528)
  line L3818 (26.916944, 289.824583) -> (26.9875, 289.789305)
  line L3819 (36.300833, 261.531805) -> (35.171944, 265.130139)
  line L3820 (36.336111, 261.390694) -> (36.300833, 261.46125)
  line L3821 (28.504444, 222.549861) -> (24.024167, 218.034306)
  line L3822 (24.024167, 218.034306) -> (19.085278, 218.034306)
  line L3823 (19.085278, 218.034306) -> (23.600833, 222.549861)
  line L3824 (23.600833, 222.549861) -> (28.504444, 222.549861)
  line L3825 (22.154444, 222.549861) -> (17.674167, 218.034306)
  line L3826 (32.984722, 289.154305) -> (33.196389, 289.260139)
  line L3827 (33.196389, 289.260139) -> (33.443333, 289.295417)
  line L3828 (15.451667, 225.301528) -> (15.204722, 225.26625)
  line L3829 (40.3225, 253.20625) -> (40.393056, 253.170972)
  line L3830 (6.173611, 223.114305) -> (6.067778, 223.114305)
  line L3831 (6.067778, 223.114305) -> (5.961944, 223.184861)
  line L3832 (10.971389, 224.595972) -> (10.900833, 224.595972)
  line L3833 (33.3375, 272.362083) -> (33.408056, 272.291528)
  line L3834 (33.408056, 272.291528) -> (33.584444, 272.25625)
  line L3835 (28.645556, 250.384028) -> (28.680833, 250.560417)
  line L3836 (28.2575, 250.560417) -> (28.292778, 250.384028)
  line L3837 (39.440556, 244.95125) -> (39.616944, 244.915972)
  line L3838 (11.606389, 233.344861) -> (11.606389, 233.732917)
  line L3839 (11.606389, 233.732917) -> (11.535833, 234.085694)
  line L3840 (11.535833, 234.085694) -> (11.43, 234.403194)
  line L3841 (37.958889, 294.763472) -> (35.983333, 294.763472)
  line L3842 (34.572222, 288.801528) -> (34.6075, 288.907361)
  line L3843 (22.013333, 225.019305) -> (21.942778, 225.019305)
  line L3844 (27.234444, 253.029861) -> (27.305, 252.88875)
  line L3845 (29.739167, 232.004305) -> (29.633333, 231.93375)
  line L3846 (40.110833, 253.170972) -> (40.181389, 253.20625)
  line L3847 (26.317222, 250.34875) -> (26.3525, 250.384028)
  line L3848 (26.3525, 250.384028) -> (26.387778, 250.560417)
  line L3849 (35.454167, 291.376805) -> (35.454167, 294.939861)
  line L3850 (38.205833, 236.449305) -> (38.241111, 236.555139)
  line L3851 (31.961667, 223.643472) -> (32.0675, 223.643472)
  line L3852 (38.840833, 243.575417) -> (38.770278, 243.751805)
  line L3853 (38.770278, 243.751805) -> (38.735, 243.928194)
  line L3854 (39.087778, 243.434305) -> (38.946667, 243.469583)
  line L3855 (38.946667, 243.469583) -> (38.840833, 243.575417)
  line L3856 (26.9875, 289.789305) -> (27.093333, 289.754028)
  line L3857 (30.127222, 253.594305) -> (30.197778, 253.594305)
  line L3858 (40.251944, 253.20625) -> (40.3225, 253.20625)
  line L3859 (13.476111, 257.615972) -> (13.335, 257.898194)
  line L3860 (38.488056, 240.788472) -> (40.075556, 240.788472)
  line L3861 (42.298056, 264.248194) -> (42.403889, 264.283472)
  line L3862 (42.403889, 264.283472) -> (42.509722, 264.354028)
  line L3863 (42.509722, 264.354028) -> (42.545, 264.459861)
  line L3864 (18.803056, 225.58375) -> (18.626667, 225.477917)
  line L3865 (38.523333, 253.065139) -> (39.299444, 251.512917)
  line L3866 (13.934722, 288.695694) -> (14.005278, 288.307639)
  line L3867 (25.011944, 289.824583) -> (25.0825, 289.789305)
  line L3868 (38.276389, 243.928194) -> (38.311667, 244.245694)
  line L3869 (26.211389, 224.31375) -> (26.176111, 224.63125)
  line L3870 (28.010556, 224.137361) -> (27.834167, 223.925694)
  line L3871 (32.737778, 238.707083) -> (32.455556, 238.177917)
  line L3872 (33.372778, 272.679583) -> (33.3375, 272.57375)
  line L3873 (33.3375, 272.57375) -> (33.302222, 272.467917)
  line L3874 (14.781389, 256.910417) -> (14.499167, 256.945694)
  line L3875 (29.280556, 251.442361) -> (29.351111, 251.442361)
  line L3876 (29.351111, 251.442361) -> (29.421667, 251.477639)
  line L3877 (34.6075, 288.907361) -> (34.642778, 288.977917)
  line L3878 (34.113611, 288.872083) -> (34.219444, 288.730972)
  line L3879 (34.6075, 287.778472) -> (34.642778, 287.637361)
  line L3880 (39.193611, 276.277917) -> (37.323889, 272.397361)
  line L3881 (39.828611, 243.892917) -> (39.828611, 243.963472)
  line L3882 (25.611667, 247.385417) -> (25.011944, 247.244305)
  line L3883 (25.011944, 247.244305) -> (24.412222, 247.032639)
  line L3884 (26.3525, 295.821805) -> (25.611667, 295.821805)
  line L3885 (43.991389, 287.390417) -> (43.991389, 288.836805)
  line L3886 (7.584722, 234.579583) -> (7.796389, 234.897083)
  line L3887 (7.796389, 234.897083) -> (8.043333, 235.144028)
  line L3888 (19.014722, 225.936528) -> (18.908889, 225.724861)
  line L3889 (38.311667, 295.11625) -> (38.276389, 295.186805)
  line L3890 (21.59, 244.669028) -> (21.942778, 245.198194)
  line L3891 (41.874722, 273.490972) -> (40.781111, 273.490972)
  line L3892 (22.436667, 284.885694) -> (27.199167, 284.885694)
  line L3893 (10.900833, 224.595972) -> (10.830278, 224.63125)
  line L3894 (12.065, 226.112917) -> (11.288889, 224.807639)
  line L3895 (33.443333, 293.352361) -> (32.526111, 293.352361)
  line L3896 (38.064722, 289.824583) -> (38.170556, 289.789305)
  line L3897 (32.279167, 287.990139) -> (32.243889, 287.707917)
  line L3898 (32.243889, 287.707917) -> (32.279167, 287.390417)
  line L3899 (29.668611, 228.75875) -> (29.598056, 228.864583)
  line L3900 (9.913056, 223.36125) -> (9.913056, 223.255417)
  line L3901 (33.055278, 246.009583) -> (32.596667, 246.53875)
  line L3902 (32.596667, 246.53875) -> (32.102778, 247.032639)
  line L3903 (32.102778, 247.032639) -> (31.573611, 247.455972)
  line L3904 (35.454167, 227.382917) -> (35.665833, 227.312361)
  line L3905 (32.0675, 295.186805) -> (32.032222, 295.080972)
  line L3906 (32.032222, 295.080972) -> (31.996944, 294.939861)
  line L3907 (33.478611, 295.292639) -> (32.385, 295.292639)
  line L3908 (31.079722, 230.416805) -> (31.115, 230.487361)
  line L3909 (31.115, 230.487361) -> (31.115, 230.557917)
  line L3910 (29.986111, 230.381528) -> (30.868056, 230.381528)
  line L3911 (40.604722, 272.961805) -> (42.051111, 272.961805)
  line L3912 (40.463611, 272.397361) -> (40.604722, 272.961805)
  line L3913 (40.216667, 272.25625) -> (40.287222, 272.25625)
  line L3914 (28.998333, 231.651528) -> (28.927778, 231.61625)
  line L3915 (39.793333, 244.034028) -> (39.828611, 243.963472)
  line L3916 (39.828611, 243.963472) -> (39.828611, 243.892917)
  line L3917 (39.37, 244.457361) -> (39.581667, 244.422083)
  line L3918 (39.581667, 244.422083) -> (39.6875, 244.31625)
  line L3919 (30.868056, 246.080139) -> (31.361944, 245.656805)
  line L3920 (24.412222, 235.285139) -> (23.847778, 235.567361)
  line L3921 (34.466389, 276.313194) -> (33.372778, 272.679583)
  line L3922 (34.713333, 276.489583) -> (34.6075, 276.489583)
  line L3923 (34.6075, 276.489583) -> (34.536944, 276.454305)
  line L3924 (27.728333, 250.384028) -> (27.763611, 250.454583)
  line L3925 (27.763611, 250.454583) -> (27.763611, 250.525139)
  line L3926 (35.454167, 291.235694) -> (35.454167, 291.376805)
  line L3927 (20.672778, 226.677361) -> (21.096111, 227.100694)
  line L3928 (21.096111, 227.100694) -> (21.413611, 227.277083)
  line L3929 (21.413611, 227.277083) -> (21.9075, 227.382917)
  line L3930 (24.729722, 285.555972) -> (24.659167, 285.59125)
  line L3931 (17.215556, 290.812361) -> (16.968611, 290.918194)
  line L3932 (16.968611, 290.918194) -> (16.721667, 291.024028)
  line L3933 (24.906111, 234.297361) -> (25.541111, 234.15625)
  line L3934 (25.541111, 234.15625) -> (26.211389, 234.085694)
  line L3935 (43.991389, 295.186805) -> (43.991389, 293.740417)
  line L3936 (14.957778, 287.108194) -> (15.310556, 286.967083)
  line L3937 (15.310556, 286.967083) -> (15.663333, 286.86125)
  line L3938 (35.771667, 291.059305) -> (35.665833, 291.059305)
  line L3939 (11.324167, 218.034306) -> (6.385278, 218.034306)
  line L3940 (6.385278, 218.034306) -> (10.900833, 222.549861)
  line L3941 (10.900833, 222.549861) -> (15.804444, 222.549861)
  line L3942 (9.454444, 222.549861) -> (4.974167, 218.034306)
  line L3943 (31.009167, 289.683472) -> (31.044444, 289.542361)
  line L3944 (26.211389, 224.31375) -> (26.387778, 223.99625)
  line L3945 (32.526111, 294.763472) -> (33.513889, 294.763472)
  line L3946 (39.581667, 243.293194) -> (39.899167, 243.187361)
  line L3947 (27.728333, 291.094583) -> (27.6225, 291.059305)
  line L3948 (8.643056, 235.532083) -> (8.995833, 235.637917)
  line L3949 (8.995833, 235.637917) -> (9.383889, 235.673194)
  line L3950 (30.832778, 295.080972) -> (30.832778, 294.975139)
  line L3951 (29.809722, 294.763472) -> (29.950833, 294.79875)
  line L3952 (32.526111, 293.352361) -> (32.526111, 294.763472)
  line L3953 (39.017222, 240.329861) -> (38.452778, 240.329861)
  line L3954 (27.481389, 247.455972) -> (28.081111, 247.385417)
  line L3955 (40.357778, 240.541528) -> (40.3225, 240.647361)
  line L3956 (40.3225, 240.647361) -> (40.251944, 240.753194)
  line L3957 (29.598056, 231.827917) -> (29.633333, 231.93375)
  line L3958 (34.536944, 287.919583) -> (34.395833, 287.990139)
  line L3959 (34.395833, 287.990139) -> (34.29, 287.990139)
  line L3960 (33.655, 287.990139) -> (33.549167, 287.990139)
  line L3961 (33.549167, 287.990139) -> (33.443333, 287.954861)
  line L3962 (23.106944, 225.195694) -> (23.106944, 224.172639)
  line L3963 (38.346944, 291.30625) -> (38.311667, 291.165139)
  line L3964 (28.116389, 224.419583) -> (28.151667, 224.807639)
  line L3965 (23.8125, 285.697083) -> (23.8125, 285.838194)
  line L3966 (7.972778, 295.821805) -> (12.911667, 295.821805)
  line L3967 (39.899167, 234.826528) -> (39.863889, 234.79125)
  line L3968 (39.017222, 237.33125) -> (39.017222, 240.329861)
  line L3969 (27.587222, 228.794028) -> (27.551944, 228.75875)
  line L3970 (31.291389, 257.01625) -> (30.973889, 256.945694)
  line L3971 (32.737778, 238.707083) -> (32.949444, 239.306805)